Autodesk Inventor part; units mm, degrees
(part 3 of 3)
sketch "Szkic15" plane through (0, 0, 0) normal (0, 0, -1) x (-1, 0, 0)
  line L0 (-9.2546, 25.2956) -> (16.7454, 25.2956) projected
  line L1 (3.7454, 25.2956) -> (3.7525, -18.7044)
  line L2 (-0.9375, -18.7044) -> (8.4425, -18.7044) projected
  circle A0 centre (3.749, 3.2956) radius 15
  line L3 (19.3551, 10.4983) -> (20.5264, 12.5271)
  line L4 (20.5264, 12.5271) -> (22.8692, 12.5271)
  line L5 (22.8692, 12.5271) -> (24.0404, 10.4983)
  line L6 (24.0404, 10.4983) -> (22.8692, 8.4695)
  line L7 (22.8692, 8.4695) -> (20.5264, 8.4695)
  line L8 (20.5264, 8.4695) -> (19.3551, 10.4983)
  line L9 (13.7752, 12.4981) -> (11.4324, 12.4981)
  line L10 (11.4324, 12.4981) -> (10.2611, 10.4693)
  line L11 (10.2611, 10.4693) -> (11.4324, 8.4405)
  line L12 (11.4324, 8.4405) -> (13.7752, 8.4405)
  line L13 (13.7752, 8.4405) -> (14.9464, 10.4693)
  line L14 (14.9464, 10.4693) -> (13.7752, 12.4981)
  line L15 (14.8161, 7.7843) -> (15.9874, 9.8131)
  line L16 (15.9874, 9.8131) -> (18.3302, 9.8131)
  line L17 (18.3302, 9.8131) -> (19.5014, 7.7843)
  line L18 (19.5014, 7.7843) -> (18.3302, 5.7555)
  line L19 (18.3302, 5.7555) -> (15.9874, 5.7555)
  line L20 (15.9874, 5.7555) -> (14.8161, 7.7843)
  line L21 (18.2702, 11.0065) -> (19.4414, 13.0353)
  line L22 (19.4414, 13.0353) -> (18.2702, 15.0641)
  line L23 (18.2702, 15.0641) -> (15.9274, 15.0641)
  line L24 (15.9274, 15.0641) -> (14.7561, 13.0353)
  line L25 (14.7561, 13.0353) -> (15.9274, 11.0065)
  line L26 (15.9274, 11.0065) -> (18.2702, 11.0065)
  line L27 (0.9421, 10.4263) -> (2.1134, 12.4551)
  line L28 (2.1134, 12.4551) -> (4.4562, 12.4551)
  line L29 (4.4562, 12.4551) -> (5.6274, 10.4263)
  line L30 (5.6274, 10.4263) -> (4.4562, 8.3975)
  line L31 (4.4562, 8.3975) -> (2.1134, 8.3975)
  line L32 (2.1134, 8.3975) -> (0.9421, 10.4263)
  line L33 (-3.5969, 7.7123) -> (-2.4256, 9.7411)
  line L34 (-2.4256, 9.7411) -> (-0.0828, 9.7411)
  line L35 (-0.0828, 9.7411) -> (1.0884, 7.7123)
  line L36 (1.0884, 7.7123) -> (-0.0828, 5.6835)
  line L37 (-0.0828, 5.6835) -> (-2.4256, 5.6835)
  line L38 (-2.4256, 5.6835) -> (-3.5969, 7.7123)
  line L39 (2.2234, 7.1181) -> (1.0521, 5.0893)
  line L40 (1.0521, 5.0893) -> (2.2234, 3.0605)
  line L41 (2.2234, 3.0605) -> (4.5662, 3.0605)
  line L42 (4.5662, 3.0605) -> (5.7374, 5.0893)
  line L43 (5.7374, 5.0893) -> (4.5662, 7.1181)
  line L44 (4.5662, 7.1181) -> (2.2234, 7.1181)
  line L45 (-3.3977, 4.9903) -> (-4.5689, 7.0191)
  line L46 (-4.5689, 7.0191) -> (-6.9117, 7.0191)
  line L47 (-6.9117, 7.0191) -> (-8.083, 4.9903)
  line L48 (-8.083, 4.9903) -> (-6.9117, 2.9615)
  line L49 (-6.9117, 2.9615) -> (-4.5689, 2.9615)
  line L50 (-4.5689, 2.9615) -> (-3.3977, 4.9903)
  line L51 (-2.2726, 4.5521) -> (-3.4439, 2.5233)
  line L52 (-3.4439, 2.5233) -> (-2.2726, 0.4945)
  line L53 (-2.2726, 0.4945) -> (0.0702, 0.4945)
  line L54 (0.0702, 0.4945) -> (1.2414, 2.5233)
  line L55 (1.2414, 2.5233) -> (0.0702, 4.5521)
  line L56 (0.0702, 4.5521) -> (-2.2726, 4.5521)
  line L57 (6.6694, 5.7115) -> (9.0122, 5.7115)
  line L58 (9.0122, 5.7115) -> (10.1834, 7.7403)
  line L59 (10.1834, 7.7403) -> (9.0122, 9.7691)
  line L60 (9.0122, 9.7691) -> (6.6694, 9.7691)
  line L61 (6.6694, 9.7691) -> (5.4981, 7.7403)
  line L62 (5.4981, 7.7403) -> (6.6694, 5.7115)
  line L63 (2.2824, 1.8671) -> (1.1111, -0.1617)
  line L64 (1.1111, -0.1617) -> (2.2824, -2.1905)
  line L65 (2.2824, -2.1905) -> (4.6252, -2.1905)
  line L66 (4.6252, -2.1905) -> (5.7964, -0.1617)
  line L67 (5.7964, -0.1617) -> (4.6252, 1.8671)
  line L68 (4.6252, 1.8671) -> (2.2824, 1.8671)
  line L69 (5.6511, 2.5523) -> (6.8224, 4.5811)
  line L70 (6.8224, 4.5811) -> (9.1652, 4.5811)
  line L71 (9.1652, 4.5811) -> (10.3364, 2.5523)
  line L72 (10.3364, 2.5523) -> (9.1652, 0.5235)
  line L73 (9.1652, 0.5235) -> (6.8224, 0.5235)
  line L74 (6.8224, 0.5235) -> (5.6511, 2.5523)
  line L75 (19.4651, 5.1613) -> (20.6364, 7.1901)
  line L76 (20.6364, 7.1901) -> (22.9792, 7.1901)
  line L77 (22.9792, 7.1901) -> (24.1504, 5.1613)
  line L78 (24.1504, 5.1613) -> (22.9792, 3.1325)
  line L79 (22.9792, 3.1325) -> (20.6364, 3.1325)
  line L80 (20.6364, 3.1325) -> (19.4651, 5.1613)
  line L81 (16.1404, 4.6241) -> (14.9691, 2.5953)
  line L82 (14.9691, 2.5953) -> (16.1404, 0.5665)
  line L83 (16.1404, 0.5665) -> (18.4832, 0.5665)
  line L84 (18.4832, 0.5665) -> (19.6544, 2.5953)
  line L85 (19.6544, 2.5953) -> (18.4832, 4.6241)
  line L86 (18.4832, 4.6241) -> (16.1404, 4.6241)
  line L87 (11.3174, 7.1461) -> (10.1461, 5.1173)
  line L88 (10.1461, 5.1173) -> (11.3174, 3.0885)
  line L89 (11.3174, 3.0885) -> (13.6602, 3.0885)
  line L90 (13.6602, 3.0885) -> (14.8314, 5.1173)
  line L91 (14.8314, 5.1173) -> (13.6602, 7.1461)
  line L92 (13.6602, 7.1461) -> (11.3174, 7.1461)
  line L93 (11.3774, 1.8961) -> (10.2061, -0.1327)
  line L94 (10.2061, -0.1327) -> (11.3774, -2.1615)
  line L95 (11.3774, -2.1615) -> (13.7202, -2.1615)
  line L96 (13.7202, -2.1615) -> (14.8914, -0.1327)
  line L97 (14.8914, -0.1327) -> (13.7202, 1.8961)
  line L98 (13.7202, 1.8961) -> (11.3774, 1.8961)
  line L99 (-3.3381, -0.2607) -> (-4.5093, 1.7681)
  line L100 (-4.5093, 1.7681) -> (-6.8521, 1.7681)
  line L101 (-6.8521, 1.7681) -> (-8.0234, -0.2607)
  line L102 (-8.0234, -0.2607) -> (-6.8521, -2.2895)
  line L103 (-6.8521, -2.2895) -> (-4.5093, -2.2895)
  line L104 (-4.5093, -2.2895) -> (-3.3381, -0.2607)
  line L105 (0.1912, -0.9189) -> (-2.1516, -0.9189)
  line L106 (-2.1516, -0.9189) -> (-3.3229, -2.9477)
  line L107 (-3.3229, -2.9477) -> (-2.1516, -4.9765)
  line L108 (-2.1516, -4.9765) -> (0.1912, -4.9765)
  line L109 (0.1912, -4.9765) -> (1.3624, -2.9477)
  line L110 (1.3624, -2.9477) -> (0.1912, -0.9189)
  line L111 (1.2761, -5.4847) -> (2.4474, -3.4559)
  line L112 (2.4474, -3.4559) -> (4.7902, -3.4559)
  line L113 (4.7902, -3.4559) -> (5.9614, -5.4847)
  line L114 (5.9614, -5.4847) -> (4.7902, -7.5135)
  line L115 (4.7902, -7.5135) -> (2.4474, -7.5135)
  line L116 (2.4474, -7.5135) -> (1.2761, -5.4847)
  line L117 (-3.1334, -5.5137) -> (-4.3046, -3.4849)
  line L118 (-4.3046, -3.4849) -> (-6.6474, -3.4849)
  line L119 (-6.6474, -3.4849) -> (-7.8187, -5.5137)
  line L120 (-7.8187, -5.5137) -> (-6.6474, -7.5425)
  line L121 (-6.6474, -7.5425) -> (-4.3046, -7.5425)
  line L122 (-4.3046, -7.5425) -> (-3.1334, -5.5137)
  line L123 (9.2852, -4.9475) -> (10.4564, -2.9187)
  line L124 (10.4564, -2.9187) -> (9.2852, -0.8899)
  line L125 (9.2852, -0.8899) -> (6.9424, -0.8899)
  line L126 (6.9424, -0.8899) -> (5.7711, -2.9187)
  line L127 (5.7711, -2.9187) -> (6.9424, -4.9475)
  line L128 (6.9424, -4.9475) -> (9.2852, -4.9475)
  line L129 (18.6042, -0.8469) -> (16.2614, -0.8469)
  line L130 (16.2614, -0.8469) -> (15.0901, -2.8757)
  line L131 (15.0901, -2.8757) -> (16.2614, -4.9045)
  line L132 (16.2614, -4.9045) -> (18.6042, -4.9045)
  line L133 (18.6042, -4.9045) -> (19.7754, -2.8757)
  line L134 (19.7754, -2.8757) -> (18.6042, -0.8469)
  line L135 (14.1082, -3.4129) -> (11.7654, -3.4129)
  line L136 (11.7654, -3.4129) -> (10.5941, -5.4417)
  line L137 (10.5941, -5.4417) -> (11.7654, -7.4705)
  line L138 (11.7654, -7.4705) -> (14.1082, -7.4705)
  line L139 (14.1082, -7.4705) -> (15.2794, -5.4417)
  line L140 (15.2794, -5.4417) -> (14.1082, -3.4129)
  line L141 (24.2094, -0.0897) -> (23.0382, 1.9391)
  line L142 (23.0382, 1.9391) -> (20.6954, 1.9391)
  line L143 (20.6954, 1.9391) -> (19.5241, -0.0897)
  line L144 (19.5241, -0.0897) -> (20.6954, -2.1185)
  line L145 (20.6954, -2.1185) -> (23.0382, -2.1185)
  line L146 (23.0382, -2.1185) -> (24.2094, -0.0897)
  line L147 (24.1841, -2.8467) -> (25.3554, -0.8179)
  line L148 (25.3554, -0.8179) -> (27.6982, -0.8179)
  line L149 (27.6982, -0.8179) -> (28.8694, -2.8467)
  line L150 (28.8694, -2.8467) -> (27.6982, -4.8755)
  line L151 (27.6982, -4.8755) -> (25.3554, -4.8755)
  line L152 (25.3554, -4.8755) -> (24.1841, -2.8467)
  line L153 (23.2032, -3.3839) -> (20.8604, -3.3839)
  line L154 (20.8604, -3.3839) -> (19.6891, -5.4127)
  line L155 (19.6891, -5.4127) -> (20.8604, -7.4415)
  line L156 (20.8604, -7.4415) -> (23.2032, -7.4415)
  line L157 (23.2032, -7.4415) -> (24.3744, -5.4127)
  line L158 (24.3744, -5.4127) -> (23.2032, -3.3839)
  line L159 (1.3851, -10.8217) -> (2.5564, -8.7929)
  line L160 (2.5564, -8.7929) -> (4.8992, -8.7929)
  line L161 (4.8992, -8.7929) -> (6.0704, -10.8217)
  line L162 (6.0704, -10.8217) -> (4.8992, -12.8505)
  line L163 (4.8992, -12.8505) -> (2.5564, -12.8505)
  line L164 (2.5564, -12.8505) -> (1.3851, -10.8217)
  line L165 (0.4042, -11.3589) -> (-1.9386, -11.3589)
  line L166 (-1.9386, -11.3589) -> (-3.1099, -13.3877)
  line L167 (-3.1099, -13.3877) -> (-1.9386, -15.4165)
  line L168 (-1.9386, -15.4165) -> (0.4042, -15.4165)
  line L169 (0.4042, -15.4165) -> (1.5754, -13.3877)
  line L170 (1.5754, -13.3877) -> (0.4042, -11.3589)
  line L171 (0.2502, -10.2275) -> (1.4214, -8.1987)
  line L172 (1.4214, -8.1987) -> (0.2502, -6.1699)
  line L173 (0.2502, -6.1699) -> (-2.0926, -6.1699)
  line L174 (-2.0926, -6.1699) -> (-3.2639, -8.1987)
  line L175 (-3.2639, -8.1987) -> (-2.0926, -10.2275)
  line L176 (-2.0926, -10.2275) -> (0.2502, -10.2275)
  line L177 (-4.2356, -8.8919) -> (-6.5784, -8.8919)
  line L178 (-6.5784, -8.8919) -> (-7.7497, -10.9207)
  line L179 (-7.7497, -10.9207) -> (-6.5784, -12.9495)
  line L180 (-6.5784, -12.9495) -> (-4.2356, -12.9495)
  line L181 (-4.2356, -12.9495) -> (-3.0644, -10.9207)
  line L182 (-3.0644, -10.9207) -> (-4.2356, -8.8919)
  line L183 (5.8311, -8.1697) -> (7.0024, -6.1409)
  line L184 (7.0024, -6.1409) -> (9.3452, -6.1409)
  line L185 (9.3452, -6.1409) -> (10.5164, -8.1697)
  line L186 (10.5164, -8.1697) -> (9.3452, -10.1985)
  line L187 (9.3452, -10.1985) -> (7.0024, -10.1985)
  line L188 (7.0024, -10.1985) -> (5.8311, -8.1697)
  line L189 (5.9841, -13.3587) -> (7.1554, -11.3299)
  line L190 (7.1554, -11.3299) -> (9.4982, -11.3299)
  line L191 (9.4982, -11.3299) -> (10.6694, -13.3587)
  line L192 (10.6694, -13.3587) -> (9.4982, -15.3875)
  line L193 (9.4982, -15.3875) -> (7.1554, -15.3875)
  line L194 (7.1554, -15.3875) -> (5.9841, -13.3587)
  line L195 (2.6164, -18.1015) -> (4.9592, -18.1015)
  line L196 (4.9592, -18.1015) -> (6.1304, -16.0727)
  line L197 (6.1304, -16.0727) -> (4.9592, -14.0439)
  line L198 (4.9592, -14.0439) -> (2.6164, -14.0439)
  line L199 (2.6164, -14.0439) -> (1.4451, -16.0727)
  line L200 (1.4451, -16.0727) -> (2.6164, -18.1015)
  line L201 (11.6514, -8.7639) -> (10.4801, -10.7927)
  line L202 (10.4801, -10.7927) -> (11.6514, -12.8215)
  line L203 (11.6514, -12.8215) -> (13.9942, -12.8215)
  line L204 (13.9942, -12.8215) -> (15.1654, -10.7927)
  line L205 (15.1654, -10.7927) -> (13.9942, -8.7639)
  line L206 (13.9942, -8.7639) -> (11.6514, -8.7639)
  line L207 (15.3031, -13.3157) -> (16.4744, -11.2869)
  line L208 (16.4744, -11.2869) -> (18.8172, -11.2869)
  line L209 (18.8172, -11.2869) -> (19.9884, -13.3157)
  line L210 (19.9884, -13.3157) -> (18.8172, -15.3445)
  line L211 (18.8172, -15.3445) -> (16.4744, -15.3445)
  line L212 (16.4744, -15.3445) -> (15.3031, -13.3157)
  line L213 (15.1491, -8.1267) -> (16.3204, -6.0979)
  line L214 (16.3204, -6.0979) -> (18.6632, -6.0979)
  line L215 (18.6632, -6.0979) -> (19.8344, -8.1267)
  line L216 (19.8344, -8.1267) -> (18.6632, -10.1555)
  line L217 (18.6632, -10.1555) -> (16.3204, -10.1555)
  line L218 (16.3204, -10.1555) -> (15.1491, -8.1267)
  line L219 (19.7981, -10.7497) -> (20.9694, -8.7209)
  line L220 (20.9694, -8.7209) -> (23.3122, -8.7209)
  line L221 (23.3122, -8.7209) -> (24.4834, -10.7497)
  line L222 (24.4834, -10.7497) -> (23.3122, -12.7785)
  line L223 (23.3122, -12.7785) -> (20.9694, -12.7785)
  line L224 (20.9694, -12.7785) -> (19.7981, -10.7497)
  line L225 (25.4154, -10.1265) -> (27.7582, -10.1265)
  line L226 (27.7582, -10.1265) -> (28.9294, -8.0977)
  line L227 (28.9294, -8.0977) -> (27.7582, -6.0689)
  line L228 (27.7582, -6.0689) -> (25.4154, -6.0689)
  line L229 (25.4154, -6.0689) -> (24.2441, -8.0977)
  line L230 (24.2441, -8.0977) -> (25.4154, -10.1265)
  line L231 (25.5684, -11.2579) -> (24.3971, -13.2867)
  line L232 (24.3971, -13.2867) -> (25.5684, -15.3155)
  line L233 (25.5684, -15.3155) -> (27.9112, -15.3155)
  line L234 (27.9112, -15.3155) -> (29.0824, -13.2867)
  line L235 (29.0824, -13.2867) -> (27.9112, -11.2579)
  line L236 (27.9112, -11.2579) -> (25.5684, -11.2579)
  line L237 (11.7104, -18.0725) -> (14.0532, -18.0725)
  line L238 (14.0532, -18.0725) -> (15.2244, -16.0437)
  line L239 (15.2244, -16.0437) -> (14.0532, -14.0149)
  line L240 (14.0532, -14.0149) -> (11.7104, -14.0149)
  line L241 (11.7104, -14.0149) -> (10.5391, -16.0437)
  line L242 (10.5391, -16.0437) -> (11.7104, -18.0725)
  line L243 (21.0294, -13.9719) -> (19.8581, -16.0007)
  line L244 (19.8581, -16.0007) -> (21.0294, -18.0295)
  line L245 (21.0294, -18.0295) -> (23.3722, -18.0295)
  line L246 (23.3722, -18.0295) -> (24.5434, -16.0007)
  line L247 (24.5434, -16.0007) -> (23.3722, -13.9719)
  line L248 (23.3722, -13.9719) -> (21.0294, -13.9719)
  line L249 (-26.4363, -0.3327) -> (-25.265, 1.6961)
  line L250 (-25.265, 1.6961) -> (-22.9222, 1.6961)
  line L251 (-22.9222, 1.6961) -> (-21.751, -0.3327)
  line L252 (-21.751, -0.3327) -> (-22.9222, -2.3615)
  line L253 (-22.9222, -2.3615) -> (-25.265, -2.3615)
  line L254 (-25.265, -2.3615) -> (-26.4363, -0.3327)
  line L255 (-18.0387, -1.0469) -> (-20.3815, -1.0469)
  line L256 (-20.3815, -1.0469) -> (-21.5528, -3.0757)
  line L257 (-21.5528, -3.0757) -> (-20.3815, -5.1045)
  line L258 (-20.3815, -5.1045) -> (-18.0387, -5.1045)
  line L259 (-18.0387, -5.1045) -> (-16.8675, -3.0757)
  line L260 (-16.8675, -3.0757) -> (-18.0387, -1.0469)
  line L261 (-22.5341, -3.6119) -> (-24.8769, -3.6119)
  line L262 (-24.8769, -3.6119) -> (-26.0482, -5.6407)
  line L263 (-26.0482, -5.6407) -> (-24.8769, -7.6695)
  line L264 (-24.8769, -7.6695) -> (-22.5341, -7.6695)
  line L265 (-22.5341, -7.6695) -> (-21.3629, -5.6407)
  line L266 (-21.3629, -5.6407) -> (-22.5341, -3.6119)
  line L267 (-27.357, -1.0899) -> (-29.6998, -1.0899)
  line L268 (-29.6998, -1.0899) -> (-30.8711, -3.1187)
  line L269 (-30.8711, -3.1187) -> (-29.6998, -5.1475)
  line L270 (-29.6998, -5.1475) -> (-27.357, -5.1475)
  line L271 (-27.357, -5.1475) -> (-26.1858, -3.1187)
  line L272 (-26.1858, -3.1187) -> (-27.357, -1.0899)
  line L273 (-16.9536, -5.6127) -> (-15.7823, -3.5839)
  line L274 (-15.7823, -3.5839) -> (-13.4395, -3.5839)
  line L275 (-13.4395, -3.5839) -> (-12.2683, -5.6127)
  line L276 (-12.2683, -5.6127) -> (-13.4395, -7.6415)
  line L277 (-13.4395, -7.6415) -> (-15.7823, -7.6415)
  line L278 (-15.7823, -7.6415) -> (-16.9536, -5.6127)
  line L279 (-27.4773, 0.3235) -> (-26.3061, 2.3523)
  line L280 (-26.3061, 2.3523) -> (-27.4773, 4.3811)
  line L281 (-27.4773, 4.3811) -> (-29.8201, 4.3811)
  line L282 (-29.8201, 4.3811) -> (-30.9914, 2.3523)
  line L283 (-30.9914, 2.3523) -> (-29.8201, 0.3235)
  line L284 (-29.8201, 0.3235) -> (-27.4773, 0.3235)
  line L285 (-30.8115, -8.3697) -> (-29.6402, -6.3409)
  line L286 (-29.6402, -6.3409) -> (-27.2974, -6.3409)
  line L287 (-27.2974, -6.3409) -> (-26.1262, -8.3697)
  line L288 (-26.1262, -8.3697) -> (-27.2974, -10.3985)
  line L289 (-27.2974, -10.3985) -> (-29.6402, -10.3985)
  line L290 (-29.6402, -10.3985) -> (-30.8115, -8.3697)
  line L291 (-21.4931, -8.3257) -> (-20.3218, -6.2969)
  line L292 (-20.3218, -6.2969) -> (-17.979, -6.2969)
  line L293 (-17.979, -6.2969) -> (-16.8078, -8.3257)
  line L294 (-16.8078, -8.3257) -> (-17.979, -10.3545)
  line L295 (-17.979, -10.3545) -> (-20.3218, -10.3545)
  line L296 (-20.3218, -10.3545) -> (-21.4931, -8.3257)
  line L297 (-21.3397, -13.5147) -> (-20.1684, -11.4859)
  line L298 (-20.1684, -11.4859) -> (-17.8256, -11.4859)
  line L299 (-17.8256, -11.4859) -> (-16.6544, -13.5147)
  line L300 (-16.6544, -13.5147) -> (-17.8256, -15.5435)
  line L301 (-17.8256, -15.5435) -> (-20.1684, -15.5435)
  line L302 (-20.1684, -15.5435) -> (-21.3397, -13.5147)
  line L303 (-22.6485, -8.9639) -> (-24.9913, -8.9639)
  line L304 (-24.9913, -8.9639) -> (-26.1626, -10.9927)
  line L305 (-26.1626, -10.9927) -> (-24.9913, -13.0215)
  line L306 (-24.9913, -13.0215) -> (-22.6485, -13.0215)
  line L307 (-22.6485, -13.0215) -> (-21.4773, -10.9927)
  line L308 (-21.4773, -10.9927) -> (-22.6485, -8.9639)
  line L309 (-27.1439, -11.5299) -> (-29.4867, -11.5299)
  line L310 (-29.4867, -11.5299) -> (-30.658, -13.5587)
  line L311 (-30.658, -13.5587) -> (-29.4867, -15.5875)
  line L312 (-29.4867, -15.5875) -> (-27.1439, -15.5875)
  line L313 (-27.1439, -15.5875) -> (-25.9727, -13.5587)
  line L314 (-25.9727, -13.5587) -> (-27.1439, -11.5299)
  line L315 (-24.9317, -14.2149) -> (-26.103, -16.2437)
  line L316 (-26.103, -16.2437) -> (-24.9317, -18.2725)
  line L317 (-24.9317, -18.2725) -> (-22.5889, -18.2725)
  line L318 (-22.5889, -18.2725) -> (-21.4177, -16.2437)
  line L319 (-21.4177, -16.2437) -> (-22.5889, -14.2149)
  line L320 (-22.5889, -14.2149) -> (-24.9317, -14.2149)
  line L321 (-30.5719, -11.0217) -> (-31.7431, -8.9929)
  line L322 (-31.7431, -8.9929) -> (-34.0859, -8.9929)
  line L323 (-34.0859, -8.9929) -> (-35.2572, -11.0217)
  line L324 (-35.2572, -11.0217) -> (-34.0859, -13.0505)
  line L325 (-34.0859, -13.0505) -> (-31.7431, -13.0505)
  line L326 (-31.7431, -13.0505) -> (-30.5719, -11.0217)
  line L327 (-31.6835, -14.2429) -> (-34.0263, -14.2429)
  line L328 (-34.0263, -14.2429) -> (-35.1976, -16.2717)
  line L329 (-35.1976, -16.2717) -> (-34.0263, -18.3005)
  line L330 (-34.0263, -18.3005) -> (-31.6835, -18.3005)
  line L331 (-31.6835, -18.3005) -> (-30.5123, -16.2717)
  line L332 (-30.5123, -16.2717) -> (-31.6835, -14.2429)
  line L333 (-9.3542, 16.3825) -> (-8.183, 18.4113)
  line L334 (-8.183, 18.4113) -> (-9.3542, 20.4401)
  line L335 (-9.3542, 20.4401) -> (-11.697, 20.4401)
  line L336 (-11.697, 20.4401) -> (-12.8683, 18.4113)
  line L337 (-12.8683, 18.4113) -> (-11.697, 16.3825)
  line L338 (-11.697, 16.3825) -> (-9.3542, 16.3825)
  line L339 (-17.2869, 10.2983) -> (-16.1156, 12.3271)
  line L340 (-16.1156, 12.3271) -> (-13.7728, 12.3271)
  line L341 (-13.7728, 12.3271) -> (-12.6016, 10.2983)
  line L342 (-12.6016, 10.2983) -> (-13.7728, 8.2695)
  line L343 (-13.7728, 8.2695) -> (-16.1156, 8.2695)
  line L344 (-16.1156, 8.2695) -> (-17.2869, 10.2983)
  line L345 (-13.0218, 23.6003) -> (-11.8505, 21.5715)
  line L346 (-11.8505, 21.5715) -> (-9.5077, 21.5715)
  line L347 (-9.5077, 21.5715) -> (-8.3365, 23.6003)
  line L348 (-8.3365, 23.6003) -> (-9.5077, 25.6291)
  line L349 (-9.5077, 25.6291) -> (-11.8505, 25.6291)
  line L350 (-11.8505, 25.6291) -> (-13.0218, 23.6003)
  line L351 (-13.0218, 23.6003) -> (-11.8505, 21.5715)
  line L352 (-16.8443, -10.9487) -> (-15.673, -8.9199)
  line L353 (-15.673, -8.9199) -> (-13.3302, -8.9199)
  line L354 (-13.3302, -8.9199) -> (-12.159, -10.9487)
  line L355 (-12.159, -10.9487) -> (-13.3302, -12.9775)
  line L356 (-13.3302, -12.9775) -> (-15.673, -12.9775)
  line L357 (-15.673, -12.9775) -> (-16.8443, -10.9487)
  line L358 (-11.5606, 5.5845) -> (-9.2178, 5.5845)
  line L359 (-9.2178, 5.5845) -> (-8.0466, 7.6133)
  line L360 (-8.0466, 7.6133) -> (-9.2178, 9.6421)
  line L361 (-9.2178, 9.6421) -> (-11.5606, 9.6421)
  line L362 (-11.5606, 9.6421) -> (-12.7319, 7.6133)
  line L363 (-12.7319, 7.6133) -> (-11.5606, 5.5845)
  line L364 (-12.5785, 2.4243) -> (-11.4072, 4.4531)
  line L365 (-11.4072, 4.4531) -> (-9.0644, 4.4531)
  line L366 (-9.0644, 4.4531) -> (-7.8932, 2.4243)
  line L367 (-7.8932, 2.4243) -> (-9.0644, 0.3955)
  line L368 (-9.0644, 0.3955) -> (-11.4072, 0.3955)
  line L369 (-11.4072, 0.3955) -> (-12.5785, 2.4243)
  line L370 (-13.6635, 2.9325) -> (-12.4923, 4.9613)
  line L371 (-12.4923, 4.9613) -> (-13.6635, 6.9901)
  line L372 (-13.6635, 6.9901) -> (-16.0063, 6.9901)
  line L373 (-16.0063, 6.9901) -> (-17.1776, 4.9613)
  line L374 (-17.1776, 4.9613) -> (-16.0063, 2.9325)
  line L375 (-16.0063, 2.9325) -> (-13.6635, 2.9325)
  line L376 (-12.2451, -13.4857) -> (-11.0738, -11.4569)
  line L377 (-11.0738, -11.4569) -> (-8.731, -11.4569)
  line L378 (-8.731, -11.4569) -> (-7.5598, -13.4857)
  line L379 (-7.5598, -13.4857) -> (-8.731, -15.5145)
  line L380 (-8.731, -15.5145) -> (-11.0738, -15.5145)
  line L381 (-11.0738, -15.5145) -> (-12.2451, -13.4857)
  line L382 (-15.6134, -18.2285) -> (-13.2706, -18.2285)
  line L383 (-13.2706, -18.2285) -> (-12.0994, -16.1997)
  line L384 (-12.0994, -16.1997) -> (-13.2706, -14.1709)
  line L385 (-13.2706, -14.1709) -> (-15.6134, -14.1709)
  line L386 (-15.6134, -14.1709) -> (-16.7847, -16.1997)
  line L387 (-16.7847, -16.1997) -> (-15.6134, -18.2285)
  line L388 (-7.6901, -16.1717) -> (-6.5188, -14.1429)
  line L389 (-6.5188, -14.1429) -> (-4.176, -14.1429)
  line L390 (-4.176, -14.1429) -> (-3.0048, -16.1717)
  line L391 (-3.0048, -16.1717) -> (-4.176, -18.2005)
  line L392 (-4.176, -18.2005) -> (-6.5188, -18.2005)
  line L393 (-6.5188, -18.2005) -> (-7.6901, -16.1717)
  line L394 (-8.9441, -1.0179) -> (-11.2869, -1.0179)
  line L395 (-11.2869, -1.0179) -> (-12.4582, -3.0467)
  line L396 (-12.4582, -3.0467) -> (-11.2869, -5.0755)
  line L397 (-11.2869, -5.0755) -> (-8.9441, -5.0755)
  line L398 (-8.9441, -5.0755) -> (-7.7729, -3.0467)
  line L399 (-7.7729, -3.0467) -> (-8.9441, -1.0179)
  line L400 (-12.3986, -8.2977) -> (-11.2273, -6.2689)
  line L401 (-11.2273, -6.2689) -> (-8.8845, -6.2689)
  line L402 (-8.8845, -6.2689) -> (-7.7133, -8.2977)
  line L403 (-7.7133, -8.2977) -> (-8.8845, -10.3265)
  line L404 (-8.8845, -10.3265) -> (-11.2273, -10.3265)
  line L405 (-11.2273, -10.3265) -> (-12.3986, -8.2977)
  line L406 (-4.7992, 13.6975) -> (-3.628, 15.7263)
  line L407 (-3.628, 15.7263) -> (-4.7992, 17.7551)
  line L408 (-4.7992, 17.7551) -> (-7.142, 17.7551)
  line L409 (-7.142, 17.7551) -> (-8.3133, 15.7263)
  line L410 (-8.3133, 15.7263) -> (-7.142, 13.6975)
  line L411 (-7.142, 13.6975) -> (-4.7992, 13.6975)
  line L412 (-8.152, 10.3973) -> (-6.9807, 12.4261)
  line L413 (-6.9807, 12.4261) -> (-4.6379, 12.4261)
  line L414 (-4.6379, 12.4261) -> (-3.4667, 10.3973)
  line L415 (-3.4667, 10.3973) -> (-4.6379, 8.3685)
  line L416 (-4.6379, 8.3685) -> (-6.9807, 8.3685)
  line L417 (-6.9807, 8.3685) -> (-8.152, 10.3973)
  line L418 (-12.4327, -0.2897) -> (-13.6039, 1.7391)
  line L419 (-13.6039, 1.7391) -> (-15.9467, 1.7391)
  line L420 (-15.9467, 1.7391) -> (-17.118, -0.2897)
  line L421 (-17.118, -0.2897) -> (-15.9467, -2.3185)
  line L422 (-15.9467, -2.3185) -> (-13.6039, -2.3185)
  line L423 (-13.6039, -2.3185) -> (-12.4327, -0.2897)
  line L424 (14.5261, 23.7703) -> (15.6974, 25.7991)
  line L425 (15.6974, 25.7991) -> (18.0402, 25.7991)
  line L426 (18.0402, 25.7991) -> (19.2114, 23.7703)
  line L427 (19.2114, 23.7703) -> (18.0402, 21.7415)
  line L428 (18.0402, 21.7415) -> (15.6974, 21.7415)
  line L429 (15.6974, 21.7415) -> (14.5261, 23.7703)
  line L430 (25.0224, 15.0921) -> (23.8511, 13.0633)
  line L431 (23.8511, 13.0633) -> (25.0224, 11.0345)
  line L432 (25.0224, 11.0345) -> (27.3652, 11.0345)
  line L433 (27.3652, 11.0345) -> (28.5364, 13.0633)
  line L434 (28.5364, 13.0633) -> (27.3652, 15.0921)
  line L435 (27.3652, 15.0921) -> (25.0224, 15.0921)
  line L436 (29.5514, 12.5511) -> (28.3801, 10.5223)
  line L437 (28.3801, 10.5223) -> (29.5514, 8.4935)
  line L438 (29.5514, 8.4935) -> (31.8942, 8.4935)
  line L439 (31.8942, 8.4935) -> (33.0654, 10.5223)
  line L440 (33.0654, 10.5223) -> (31.8942, 12.5511)
  line L441 (31.8942, 12.5511) -> (29.5514, 12.5511)
  line L442 (37.5604, 13.0883) -> (36.3892, 15.1171)
  line L443 (36.3892, 15.1171) -> (34.0464, 15.1171)
  line L444 (34.0464, 15.1171) -> (32.8751, 13.0883)
  line L445 (32.8751, 13.0883) -> (34.0464, 11.0595)
  line L446 (34.0464, 11.0595) -> (36.3892, 11.0595)
  line L447 (36.3892, 11.0595) -> (37.5604, 13.0883)
  line L448 (15.8504, 20.6111) -> (14.6791, 18.5823)
  line L449 (14.6791, 18.5823) -> (15.8504, 16.5535)
  line L450 (15.8504, 16.5535) -> (18.1932, 16.5535)
  line L451 (18.1932, 16.5535) -> (19.3644, 18.5823)
  line L452 (19.3644, 18.5823) -> (18.1932, 20.6111)
  line L453 (18.1932, 20.6111) -> (15.8504, 20.6111)
  line L454 (32.9351, 7.8373) -> (34.1064, 9.8661)
  line L455 (34.1064, 9.8661) -> (36.4492, 9.8661)
  line L456 (36.4492, 9.8661) -> (37.6204, 7.8373)
  line L457 (37.6204, 7.8373) -> (36.4492, 5.8085)
  line L458 (36.4492, 5.8085) -> (34.1064, 5.8085)
  line L459 (34.1064, 5.8085) -> (32.9351, 7.8373)
  line L460 (32.0732, 7.2191) -> (29.7304, 7.2191)
  line L461 (29.7304, 7.2191) -> (28.5591, 5.1903)
  line L462 (28.5591, 5.1903) -> (29.7304, 3.1615)
  line L463 (29.7304, 3.1615) -> (32.0732, 3.1615)
  line L464 (32.0732, 3.1615) -> (33.2444, 5.1903)
  line L465 (33.2444, 5.1903) -> (32.0732, 7.2191)
  line L466 (32.1332, 1.9681) -> (29.7904, 1.9681)
  line L467 (29.7904, 1.9681) -> (28.6191, -0.0607)
  line L468 (28.6191, -0.0607) -> (29.7904, -2.0895)
  line L469 (29.7904, -2.0895) -> (32.1332, -2.0895)
  line L470 (32.1332, -2.0895) -> (33.3044, -0.0607)
  line L471 (33.3044, -0.0607) -> (32.1332, 1.9681)
  line L472 (33.0881, 2.6493) -> (34.2594, 4.6781)
  line L473 (34.2594, 4.6781) -> (36.6022, 4.6781)
  line L474 (36.6022, 4.6781) -> (37.7734, 2.6493)
  line L475 (37.7734, 2.6493) -> (36.6022, 0.6205)
  line L476 (36.6022, 0.6205) -> (34.2594, 0.6205)
  line L477 (34.2594, 0.6205) -> (33.0881, 2.6493)
  line L478 (24.0641, 2.6243) -> (25.2354, 4.6531)
  line L479 (25.2354, 4.6531) -> (27.5782, 4.6531)
  line L480 (27.5782, 4.6531) -> (28.7494, 2.6243)
  line L481 (28.7494, 2.6243) -> (27.5782, 0.5955)
  line L482 (27.5782, 0.5955) -> (25.2354, 0.5955)
  line L483 (25.2354, 0.5955) -> (24.0641, 2.6243)
  line L484 (30.1234, -18.0005) -> (32.4662, -18.0005)
  line L485 (32.4662, -18.0005) -> (33.6374, -15.9717)
  line L486 (33.6374, -15.9717) -> (32.4662, -13.9429)
  line L487 (32.4662, -13.9429) -> (30.1234, -13.9429)
  line L488 (30.1234, -13.9429) -> (28.9521, -15.9717)
  line L489 (28.9521, -15.9717) -> (30.1234, -18.0005)
  line L490 (28.7131, -5.3877) -> (29.8844, -3.3589)
  line L491 (29.8844, -3.3589) -> (32.2272, -3.3589)
  line L492 (32.2272, -3.3589) -> (33.3984, -5.3877)
  line L493 (33.3984, -5.3877) -> (32.2272, -7.4165)
  line L494 (32.2272, -7.4165) -> (29.8844, -7.4165)
  line L495 (29.8844, -7.4165) -> (28.7131, -5.3877)
  line L496 (32.4072, -12.7495) -> (33.5784, -10.7207)
  line L497 (33.5784, -10.7207) -> (32.4072, -8.6919)
  line L498 (32.4072, -8.6919) -> (30.0644, -8.6919)
  line L499 (30.0644, -8.6919) -> (28.8931, -10.7207)
  line L500 (28.8931, -10.7207) -> (30.0644, -12.7495)
  line L501 (30.0644, -12.7495) -> (32.4072, -12.7495)
  line L502 (23.9101, 7.8133) -> (25.0814, 9.8421)
  line L503 (25.0814, 9.8421) -> (27.4242, 9.8421)
  line L504 (27.4242, 9.8421) -> (28.5954, 7.8133)
  line L505 (28.5954, 7.8133) -> (27.4242, 5.7845)
  line L506 (27.4242, 5.7845) -> (25.0814, 5.7845)
  line L507 (25.0814, 5.7845) -> (23.9101, 7.8133)
  line L508 (33.2681, -8.0727) -> (34.4394, -6.0439)
  line L509 (34.4394, -6.0439) -> (36.7822, -6.0439)
  line L510 (36.7822, -6.0439) -> (37.9534, -8.0727)
  line L511 (37.9534, -8.0727) -> (36.7822, -10.1015)
  line L512 (36.7822, -10.1015) -> (34.4394, -10.1015)
  line L513 (34.4394, -10.1015) -> (33.2681, -8.0727)
  line L514 (34.5934, -11.2329) -> (33.4221, -13.2617)
  line L515 (33.4221, -13.2617) -> (34.5934, -15.2905)
  line L516 (34.5934, -15.2905) -> (36.9362, -15.2905)
  line L517 (36.9362, -15.2905) -> (38.1074, -13.2617)
  line L518 (38.1074, -13.2617) -> (36.9362, -11.2329)
  line L519 (36.9362, -11.2329) -> (34.5934, -11.2329)
  line L520 (33.2091, -2.8227) -> (34.3804, -0.7939)
  line L521 (34.3804, -0.7939) -> (36.7232, -0.7939)
  line L522 (36.7232, -0.7939) -> (37.8944, -2.8227)
  line L523 (37.8944, -2.8227) -> (36.7232, -4.8515)
  line L524 (36.7232, -4.8515) -> (34.3804, -4.8515)
  line L525 (34.3804, -4.8515) -> (33.2091, -2.8227)
  line L526 (4.3362, 13.7955) -> (5.5074, 15.8243)
  line L527 (5.5074, 15.8243) -> (4.3362, 17.8531)
  line L528 (4.3362, 17.8531) -> (1.9934, 17.8531)
  line L529 (1.9934, 17.8531) -> (0.8221, 15.8243)
  line L530 (0.8221, 15.8243) -> (1.9934, 13.7955)
  line L531 (1.9934, 13.7955) -> (4.3362, 13.7955)
  line L532 (10.1234, 12.9913) -> (8.9522, 15.0201)
  line L533 (8.9522, 15.0201) -> (6.6094, 15.0201)
  line L534 (6.6094, 15.0201) -> (5.4381, 12.9913)
  line L535 (5.4381, 12.9913) -> (6.6094, 10.9625)
  line L536 (6.6094, 10.9625) -> (8.9522, 10.9625)
  line L537 (8.9522, 10.9625) -> (10.1234, 12.9913)
  line L538 (-3.7339, 18.5103) -> (-2.5626, 20.5391)
  line L539 (-2.5626, 20.5391) -> (-0.2198, 20.5391)
  line L540 (-0.2198, 20.5391) -> (0.9514, 18.5103)
  line L541 (0.9514, 18.5103) -> (-0.2198, 16.4815)
  line L542 (-0.2198, 16.4815) -> (-2.5626, 16.4815)
  line L543 (-2.5626, 16.4815) -> (-3.7339, 18.5103)
  line L544 (-0.1428, 14.9921) -> (-2.4856, 14.9921)
  line L545 (-2.4856, 14.9921) -> (-3.6569, 12.9633)
  line L546 (-3.6569, 12.9633) -> (-2.4856, 10.9345)
  line L547 (-2.4856, 10.9345) -> (-0.1428, 10.9345)
  line L548 (-0.1428, 10.9345) -> (1.0284, 12.9633)
  line L549 (1.0284, 12.9633) -> (-0.1428, 14.9921)
  line L550 (10.0464, 18.5383) -> (8.8752, 20.5671)
  line L551 (8.8752, 20.5671) -> (6.5324, 20.5671)
  line L552 (6.5324, 20.5671) -> (5.3611, 18.5383)
  line L553 (5.3611, 18.5383) -> (6.5324, 16.5095)
  line L554 (6.5324, 16.5095) -> (8.8752, 16.5095)
  line L555 (8.8752, 16.5095) -> (10.0464, 18.5383)
  line L556 (9.8571, 21.1043) -> (11.0284, 23.1331)
  line L557 (11.0284, 23.1331) -> (13.3712, 23.1331)
  line L558 (13.3712, 23.1331) -> (14.5424, 21.1043)
  line L559 (14.5424, 21.1043) -> (13.3712, 19.0755)
  line L560 (13.3712, 19.0755) -> (11.0284, 19.0755)
  line L561 (11.0284, 19.0755) -> (9.8571, 21.1043)
  line L562 (9.9161, 15.8533) -> (11.0874, 17.8821)
  line L563 (11.0874, 17.8821) -> (13.4302, 17.8821)
  line L564 (13.4302, 17.8821) -> (14.6014, 15.8533)
  line L565 (14.6014, 15.8533) -> (13.4302, 13.8245)
  line L566 (13.4302, 13.8245) -> (11.0874, 13.8245)
  line L567 (11.0874, 13.8245) -> (9.9161, 15.8533)
  line L568 (-0.3728, 21.6695) -> (0.7984, 23.6983)
  line L569 (0.7984, 23.6983) -> (-0.3728, 25.7271)
  line L570 (-0.3728, 25.7271) -> (-2.7156, 25.7271)
  line L571 (-2.7156, 25.7271) -> (-3.8869, 23.6983)
  line L572 (-3.8869, 23.6983) -> (-2.7156, 21.6695)
  line L573 (-2.7156, 21.6695) -> (-0.3728, 21.6695)
  line L574 (1.9334, 19.0465) -> (4.2762, 19.0465)
  line L575 (4.2762, 19.0465) -> (5.4474, 21.0753)
  line L576 (5.4474, 21.0753) -> (4.2762, 23.1041)
  line L577 (4.2762, 23.1041) -> (1.9334, 23.1041)
  line L578 (1.9334, 23.1041) -> (0.7621, 21.0753)
  line L579 (0.7621, 21.0753) -> (1.9334, 19.0465)
  line L580 (8.7222, 21.6985) -> (9.8934, 23.7273)
  line L581 (9.8934, 23.7273) -> (8.7222, 25.7561)
  line L582 (8.7222, 25.7561) -> (6.3794, 25.7561)
  line L583 (6.3794, 25.7561) -> (5.2081, 23.7273)
  line L584 (5.2081, 23.7273) -> (6.3794, 21.6985)
  line L585 (6.3794, 21.6985) -> (8.7222, 21.6985)
  line L586 (-3.6876, 20.9773) -> (-4.8588, 23.0061)
  line L587 (-4.8588, 23.0061) -> (-7.2016, 23.0061)
  line L588 (-7.2016, 23.0061) -> (-8.3729, 20.9773)
  line L589 (-8.3729, 20.9773) -> (-7.2016, 18.9485)
  line L590 (-7.2016, 18.9485) -> (-4.8588, 18.9485)
  line L591 (-4.8588, 18.9485) -> (-3.6876, 20.9773)
  line L592 (-22.8674, 12.2981) -> (-25.2102, 12.2981)
  line L593 (-25.2102, 12.2981) -> (-26.3815, 10.2693)
  line L594 (-26.3815, 10.2693) -> (-25.2102, 8.2405)
  line L595 (-25.2102, 8.2405) -> (-22.8674, 8.2405)
  line L596 (-22.8674, 8.2405) -> (-21.6962, 10.2693)
  line L597 (-21.6962, 10.2693) -> (-22.8674, 12.2981)
  line L598 (-20.5017, 4.4251) -> (-21.673, 2.3963)
  line L599 (-21.673, 2.3963) -> (-20.5017, 0.3675)
  line L600 (-20.5017, 0.3675) -> (-18.1589, 0.3675)
  line L601 (-18.1589, 0.3675) -> (-16.9877, 2.3963)
  line L602 (-16.9877, 2.3963) -> (-18.1589, 4.4251)
  line L603 (-18.1589, 4.4251) -> (-20.5017, 4.4251)
  line L604 (-20.6552, 9.6131) -> (-21.8265, 7.5843)
  line L605 (-21.8265, 7.5843) -> (-20.6552, 5.5555)
  line L606 (-20.6552, 5.5555) -> (-18.3124, 5.5555)
  line L607 (-18.3124, 5.5555) -> (-17.1412, 7.5843)
  line L608 (-17.1412, 7.5843) -> (-18.3124, 9.6131)
  line L609 (-18.3124, 9.6131) -> (-20.6552, 9.6131)
  line L610 (-22.9819, 6.9471) -> (-25.3247, 6.9471)
  line L611 (-25.3247, 6.9471) -> (-26.496, 4.9183)
  line L612 (-26.496, 4.9183) -> (-25.3247, 2.8895)
  line L613 (-25.3247, 2.8895) -> (-22.9819, 2.8895)
  line L614 (-22.9819, 2.8895) -> (-21.8107, 4.9183)
  line L615 (-21.8107, 4.9183) -> (-22.9819, 6.9471)
  line L616 (-29.9735, 9.5701) -> (-31.1448, 7.5413)
  line L617 (-31.1448, 7.5413) -> (-29.9735, 5.5125)
  line L618 (-29.9735, 5.5125) -> (-27.6307, 5.5125)
  line L619 (-27.6307, 5.5125) -> (-26.4595, 7.5413)
  line L620 (-26.4595, 7.5413) -> (-27.6307, 9.5701)
  line L621 (-27.6307, 9.5701) -> (-29.9735, 9.5701)
  line L622 (-27.6903, 10.7635) -> (-26.5191, 12.7923)
  line L623 (-26.5191, 12.7923) -> (-27.6903, 14.8211)
  line L624 (-27.6903, 14.8211) -> (-30.0331, 14.8211)
  line L625 (-30.0331, 14.8211) -> (-31.2044, 12.7923)
  line L626 (-31.2044, 12.7923) -> (-30.0331, 10.7635)
  line L627 (-30.0331, 10.7635) -> (-27.6903, 10.7635)
  line L628 (-20.7148, 14.8641) -> (-21.8861, 12.8353)
  line L629 (-21.8861, 12.8353) -> (-20.7148, 10.8065)
  line L630 (-20.7148, 10.8065) -> (-18.372, 10.8065)
  line L631 (-18.372, 10.8065) -> (-17.2008, 12.8353)
  line L632 (-17.2008, 12.8353) -> (-18.372, 14.8641)
  line L633 (-18.372, 14.8641) -> (-20.7148, 14.8641)
  line L634 (-3.0329, -18.9347) -> (-1.8616, -16.9059)
  line L635 (-1.8616, -16.9059) -> (0.4812, -16.9059)
  line L636 (0.4812, -16.9059) -> (1.6524, -18.9347)
  line L637 (6.0611, -18.9057) -> (7.2324, -16.8769)
  line L638 (7.2324, -16.8769) -> (9.5752, -16.8769)
  line L639 (9.5752, -16.8769) -> (10.7464, -18.9057)
  line L640 (15.3791, -18.8627) -> (16.5504, -16.8339)
  line L641 (16.5504, -16.8339) -> (18.8932, -16.8339)
  line L642 (18.8932, -16.8339) -> (20.0644, -18.8627)
  line L643 (-32.0168, 1.6671) -> (-30.8456, -0.3617)
  line L644 (-30.8456, -0.3617) -> (-32.0168, -2.3905)
  line L645 (-31.8524, -3.6559) -> (-30.6812, -5.6847)
  line L646 (-30.6812, -5.6847) -> (-31.8524, -7.7135)
  line L647 (-31.8524, -7.7135) -> (-34.1952, -7.7135)
  line L648 (-36.2385, -11.5579) -> (-35.0673, -13.5867)
  line L649 (-35.0673, -13.5867) -> (-36.2385, -15.6155)
  line L650 (-21.2629, -19.0617) -> (-20.0916, -17.0329)
  line L651 (-20.0916, -17.0329) -> (-17.7488, -17.0329)
  line L652 (-17.7488, -17.0329) -> (-16.5776, -19.0617)
  line L653 (-30.5812, -19.1057) -> (-29.4099, -17.0769)
  line L654 (-29.4099, -17.0769) -> (-27.0671, -17.0769)
  line L655 (-27.0671, -17.0769) -> (-25.8959, -19.1057)
  line L656 (-13.8938, 17.7261) -> (-12.7226, 15.6973)
  line L657 (-12.7226, 15.6973) -> (-13.8938, 13.6685)
  line L658 (-13.8938, 13.6685) -> (-16.2366, 13.6685)
  line L659 (-16.2366, 13.6685) -> (-17.4079, 15.6973)
  line L660 (-12.1683, -19.0327) -> (-10.997, -17.0039)
  line L661 (-10.997, -17.0039) -> (-8.6542, -17.0039)
  line L662 (-8.6542, -17.0039) -> (-7.483, -19.0327)
  line L663 (20.3464, 19.1185) -> (19.1751, 21.1473)
  line L664 (19.1751, 21.1473) -> (20.3464, 23.1761)
  line L665 (33.0144, 15.9253) -> (31.8432, 13.8965)
  line L666 (31.8432, 13.8965) -> (29.5004, 13.8965)
  line L667 (29.5004, 13.8965) -> (28.3291, 15.9253)
  line L668 (23.9194, 15.8973) -> (22.7482, 13.8685)
  line L669 (22.7482, 13.8685) -> (20.4054, 13.8685)
  line L670 (20.4054, 13.8685) -> (19.2341, 15.8973)
  line L671 (19.2341, 15.8973) -> (20.4054, 17.9261)
  line L672 (38.6464, 8.5225) -> (37.4751, 10.5513)
  line L673 (37.4751, 10.5513) -> (38.6464, 12.5801)
  line L674 (24.4741, -18.8337) -> (25.6454, -16.8049)
  line L675 (25.6454, -16.8049) -> (27.9882, -16.8049)
  line L676 (27.9882, -16.8049) -> (29.1594, -18.8337)
  line L677 (38.8144, -2.0645) -> (37.6431, -0.0357)
  line L678 (37.6431, -0.0357) -> (38.8144, 1.9931)
  line L679 (38.7554, 3.1855) -> (37.5841, 5.2143)
  line L680 (37.5841, 5.2143) -> (38.7554, 7.2431)
  line L681 (38.9794, -7.3885) -> (37.8081, -5.3597)
  line L682 (37.8081, -5.3597) -> (38.9794, -3.3309)
  line L683 (39.0884, -12.7245) -> (37.9171, -10.6957)
  line L684 (37.9171, -10.6957) -> (39.0884, -8.6669)
  line L685 (39.1484, -17.9755) -> (37.9771, -15.9467)
  line L686 (37.9771, -15.9467) -> (39.1484, -13.9179)
  line L687 (33.4991, -18.8087) -> (34.6704, -16.7799)
  line L688 (34.6704, -16.7799) -> (37.0132, -16.7799)
  line L689 (37.0132, -16.7799) -> (38.1844, -18.8087)
  line L690 (-22.0409, 15.6543) -> (-23.2121, 13.6255)
  line L691 (-23.2121, 13.6255) -> (-25.5549, 13.6255)
  line L692 (-25.5549, 13.6255) -> (-26.7262, 15.6543)
  line L693 (-32.0764, 6.9181) -> (-30.9052, 4.8893)
  line L694 (-30.9052, 4.8893) -> (-32.0764, 2.8605)
  line L695 (-32.1858, 12.2551) -> (-31.0146, 10.2263)
  line L696 (-31.0146, 10.2263) -> (-32.1858, 8.1975)
  line L697 (2.7374, -19.4429) -> (5.0802, -19.4429)
  line L698 (12.0554, -19.3999) -> (14.3982, -19.3999)
  line L699 (21.1504, -19.3709) -> (23.4932, -19.3709)
  line L700 (-35.2208, -8.3987) -> (-36.392, -10.4275)
  line L701 (-36.1617, -17.1049) -> (-34.9905, -19.1337)
  line L702 (-9.2774, 10.8355) -> (-11.6202, 10.8355)
  line L703 (-8.1062, 12.8643) -> (-9.2774, 10.8355)
  line L704 (-9.2774, 14.8931) -> (-8.1062, 12.8643)
  line L705 (-11.6202, 10.8355) -> (-12.7915, 12.8643)
  line L706 (-12.7915, 12.8643) -> (-11.6202, 14.8931)
  line L707 (-11.6202, 14.8931) -> (-9.2774, 14.8931)
  line L708 (13.4852, 24.4265) -> (11.1424, 24.4265)
  line L709 (27.2882, 16.5815) -> (24.9454, 16.5815)
  line L710 (36.3132, 16.6065) -> (33.9704, 16.6065)
  line L711 (38.5254, 13.9215) -> (37.3541, 15.9503)
  line L712 (30.1744, -19.3459) -> (32.5172, -19.3459)
  line L713 (4.1672, 24.3835) -> (1.8244, 24.3835)
  line L714 (-4.9278, 24.3545) -> (-7.2706, 24.3545)
  line L715 (-18.4488, 16.3535) -> (-20.7916, 16.3535)
  line L716 (-27.7672, 16.3105) -> (-30.11, 16.3105)
  line L717 (-31.1355, 15.6253) -> (-32.3067, 13.5965)
  line L718 (38.8144, -18.445) -> (-31.7211, -18.445)
  line L719 (-31.7211, -18.445) -> (-31.7211, 14.6109)
  line L720 (-12.475, 22.6532) -> (20.0445, 22.6532)
  line L721 (38.8144, 14.4269) -> (38.8144, -18.445)
  line L722 (18.6466, 14.4269) -> (36.1466, 14.4269)
  line L723 (20.0445, 22.6532) -> (19.4229, 22.6532)
  line L724 (19.4229, 22.6532) -> (19.4229, 14.4269)
  line L725 (19.4229, 14.4269) -> (38.8144, 14.4269)
  line L726 (-28.8534, 14.4269) -> (-11.3534, 14.4269)
  line L727 (-12.475, 22.6532) -> (-11.8894, 22.6532)
  line L728 (-11.8894, 22.6532) -> (-11.8894, 14.4269)
  line L729 (-11.8894, 14.4269) -> (-31.7211, 14.4269)
  line L730 (-31.7211, 14.4269) -> (-31.7211, 14.6109)
  line L731 (-11.8894, 22.6532) -> (19.4229, 22.6532)
  line L732 (19.4229, 22.6532) -> (19.4229, -18.445)
  line L733 (19.4229, -18.445) -> (-11.8894, -18.445)
  line L734 (-11.8894, -18.445) -> (-11.8894, 22.6532)
  line L735 (3.7668, 22.6532) -> (3.7668, -26.366)
  point P0 (0, 0)
  dimension "d58" = 30
  constraints: 1468 end point, 14 point on line, 5 midpoint, 2 parallel, 1 centre point, 1 horizontal, 1 perpendicular, 1 vertical
  measures "d58" diameter of A0
extrude "Wyciągnięcie proste10" cut sketch "Szkic15" against normal blind 3 contours L75 L76 L77 L78 L79 L80 | L146 L145 L144 L143 L142 L141 | L147 L148 L149 L150 L151 L152 | L158 L157 L156 L155 L154 L153 | L219 L220 L221 L222 L223 L224 | L230 L229 L228 L227 L226 L225 | L236 L235 L234 L233 L232 L231 | L249 L250 L251 L252 L253 L254 | L260 L259 L258 L257 L256 L255 | L266 L265 L264 L263 L262 L261 | L272 L271 L270 L269 L268 L267 | L273 L274 L275 L276 L277 L278 | L284 L283 L282 L281 L280 L279 | L285 L286 L287 L288 L289 L290 | L291 L292 L293 L294 L295 L296 | L297 L298 L299 L300 L301 L302 | L308 L307 L306 L305 L304 L303 | L314 L313 L312 L311 L310 L309 | L352 L353 L354 L355 L356 L357 | L375 L374 L373 L372 L371 L370 | L423 L422 L421 L420 L419 L418 | L441 L440 L439 L438 L437 L436 | L454 L455 L456 L457 L458 L459 | L465 L464 L463 L462 L461 L460 | L471 L470 L469 L468 L467 L466 | L472 L473 L474 L475 L476 L477 | L478 L479 L480 L481 L482 L483 | L490 L491 L492 L493 L494 L495 | L501 L500 L499 L498 L497 L496 | L502 L503 L504 L505 L506 L507 | L508 L509 L510 L511 L512 L513 | L519 L518 L517 L516 L515 L514 | L520 L521 L522 L523 L524 L525 | L597 L596 L595 L594 L593 L592 | L603 L602 L601 L600 L599 L598 | L609 L608 L607 L606 L605 L604 | L615 L614 L613 L612 L611 L610 | L621 L620 L619 L618 L617 L616
sketch "Szkic16" plane through (-32.7454, 17.1956, -2) normal (0, 0, -1) x (-1, 0, 0)
  arc A0 (0, 0) -> (0, -1.8) centre (0, -0.9) ccw projected
  line L0 (0, -0.9) -> (4.5, -0.9) construction
  line L1 (4.5, -1.8) -> (0, -1.8) projected
  line L2 (0, -1.5) -> (4.5, -1.5)
  line L3 (4.5, -0.3) -> (0, -0.3)
  arc A1 (0, -0.3) -> (0, -1.5) centre (0, -0.9) ccw
  arc A2 (4.5, -1.5) -> (4.5, -0.3) centre (4.5, -0.9) ccw
  line L4 (0, -0.9) -> (4.5, -0.9) construction
  line L5 (0, -1.8) -> (4.5, -1.8)
  line L6 (4.5, 0) -> (0, 0)
  arc A3 (0, 0) -> (0, -1.8) centre (0, -0.9) ccw
  arc A4 (4.5, -1.8) -> (4.5, 0) centre (4.5, -0.9) ccw
  arc A5 (9.4, -4.9) -> (7.6, -4.9) centre (8.5, -4.9) ccw projected
  arc A6 (7.6, -9.4) -> (9.4, -9.4) centre (8.5, -9.4) ccw projected
  line L7 (8.5, -4.9) -> (8.5, -9.4) construction
  line L8 (7.9, -4.9) -> (7.9, -9.4)
  line L9 (9.1, -9.4) -> (9.1, -4.9)
  arc A7 (9.1, -4.9) -> (7.9, -4.9) centre (8.5, -4.9) ccw
  arc A8 (7.9, -9.4) -> (9.1, -9.4) centre (8.5, -9.4) ccw
  line L10 (8.5, -9.4) -> (8.5, -4.9) construction
  line L11 (9.4, -9.4) -> (9.4, -4.9)
  line L12 (7.6, -4.9) -> (7.6, -9.4)
  arc A9 (7.6, -9.4) -> (9.4, -9.4) centre (8.5, -9.4) ccw
  arc A10 (9.4, -4.9) -> (7.6, -4.9) centre (8.5, -4.9) ccw
  line L13 (-33.69, 6.85) -> (-24.31, 6.85) projected
  line L14 (-29, 6.85) -> (-29, 3.0576)
  line L15 (8.5, -12.4) -> (8.5, -24.4) projected
  line L16 (8.5, -18.4) -> (5.4, -18.4)
  arc A11 (0, -35) -> (0, -36.8) centre (0, -35.9) ccw
  line L17 (0, -35.9) -> (4.5, -35.9) construction
  line L18 (4.5, -35) -> (0, -35)
  line L19 (0, -35.3) -> (4.5, -35.3)
  line L20 (4.5, -36.5) -> (0, -36.5)
  arc A12 (0, -35.3) -> (0, -36.5) centre (0, -35.9) ccw
  arc A13 (4.5, -36.5) -> (4.5, -35.3) centre (4.5, -35.9) ccw
  line L21 (0, -35.9) -> (4.5, -35.9) construction
  line L22 (0, -35) -> (4.5, -35)
  line L23 (4.5, -36.8) -> (0, -36.8)
  arc A14 (0, -35) -> (0, -36.8) centre (0, -35.9) ccw
  arc A15 (4.5, -36.8) -> (4.5, -35) centre (4.5, -35.9) ccw
  arc A16 (7.6, -31.9) -> (9.4, -31.9) centre (8.5, -31.9) ccw
  arc A17 (9.4, -27.4) -> (7.6, -27.4) centre (8.5, -27.4) ccw
  line L24 (8.5, -31.9) -> (8.5, -27.4) construction
  line L25 (7.9, -31.9) -> (7.9, -27.4)
  line L26 (9.1, -27.4) -> (9.1, -31.9)
  arc A18 (7.9, -31.9) -> (9.1, -31.9) centre (8.5, -31.9) ccw
  arc A19 (9.1, -27.4) -> (7.9, -27.4) centre (8.5, -27.4) ccw
  line L27 (8.5, -27.4) -> (8.5, -31.9) construction
  line L28 (9.4, -27.4) -> (9.4, -31.9)
  line L29 (7.6, -31.9) -> (7.6, -27.4)
  arc A20 (9.4, -27.4) -> (7.6, -27.4) centre (8.5, -27.4) ccw
  arc A21 (7.6, -31.9) -> (9.4, -31.9) centre (8.5, -31.9) ccw
  arc A22 (-58, -1.8) -> (-58, 0) centre (-58, -0.9) ccw
  line L30 (-58, -0.9) -> (-62.5, -0.9) construction
  line L31 (-62.5, -1.8) -> (-58, -1.8)
  line L32 (-58, -1.5) -> (-62.5, -1.5)
  line L33 (-62.5, -0.3) -> (-58, -0.3)
  arc A23 (-58, -1.5) -> (-58, -0.3) centre (-58, -0.9) ccw
  arc A24 (-62.5, -0.3) -> (-62.5, -1.5) centre (-62.5, -0.9) ccw
  line L34 (-58, -0.9) -> (-62.5, -0.9) construction
  line L35 (-58, -1.8) -> (-62.5, -1.8)
  line L36 (-62.5, 0) -> (-58, 0)
  arc A25 (-58, -1.8) -> (-58, 0) centre (-58, -0.9) ccw
  arc A26 (-62.5, 0) -> (-62.5, -1.8) centre (-62.5, -0.9) ccw
  arc A27 (-65.6, -4.9) -> (-67.4, -4.9) centre (-66.5, -4.9) ccw
  arc A28 (-67.4, -9.4) -> (-65.6, -9.4) centre (-66.5, -9.4) ccw
  line L37 (-66.5, -4.9) -> (-66.5, -9.4) construction
  line L38 (-65.9, -4.9) -> (-65.9, -9.4)
  line L39 (-67.1, -9.4) -> (-67.1, -4.9)
  arc A29 (-65.9, -4.9) -> (-67.1, -4.9) centre (-66.5, -4.9) ccw
  arc A30 (-67.1, -9.4) -> (-65.9, -9.4) centre (-66.5, -9.4) ccw
  line L40 (-66.5, -9.4) -> (-66.5, -4.9) construction
  line L41 (-67.4, -9.4) -> (-67.4, -4.9)
  line L42 (-65.6, -4.9) -> (-65.6, -9.4)
  arc A31 (-67.4, -9.4) -> (-65.6, -9.4) centre (-66.5, -9.4) ccw
  arc A32 (-65.6, -4.9) -> (-67.4, -4.9) centre (-66.5, -4.9) ccw
  arc A33 (-58, -36.8) -> (-58, -35) centre (-58, -35.9) ccw
  line L43 (-58, -35.9) -> (-62.5, -35.9) construction
  line L44 (-62.5, -35) -> (-58, -35)
  line L45 (-58, -35.3) -> (-62.5, -35.3)
  line L46 (-62.5, -36.5) -> (-58, -36.5)
  arc A34 (-58, -36.5) -> (-58, -35.3) centre (-58, -35.9) ccw
  arc A35 (-62.5, -35.3) -> (-62.5, -36.5) centre (-62.5, -35.9) ccw
  arc A36 (-62.5, -35) -> (-62.5, -36.8) centre (-62.5, -35.9) ccw
  line L47 (-58, -35) -> (-62.5, -35)
  line L48 (-58, -35.9) -> (-62.5, -35.9) construction
  line L49 (-62.5, -36.8) -> (-58, -36.8)
  arc A37 (-58, -36.8) -> (-58, -35) centre (-58, -35.9) ccw
  arc A38 (-67.1, -31.9) -> (-65.9, -31.9) centre (-66.5, -31.9) ccw
  arc A39 (-67.4, -31.9) -> (-65.6, -31.9) centre (-66.5, -31.9) ccw
  arc A40 (-67.4, -31.9) -> (-65.6, -31.9) centre (-66.5, -31.9) ccw
  line L50 (-65.6, -31.9) -> (-65.6, -27.4)
  line L51 (-65.9, -31.9) -> (-65.9, -27.4)
  line L52 (-66.5, -31.9) -> (-66.5, -27.4) construction
  line L53 (-66.5, -27.4) -> (-66.5, -31.9) construction
  line L54 (-67.1, -27.4) -> (-67.1, -31.9)
  line L55 (-67.4, -27.4) -> (-67.4, -31.9)
  arc A41 (-65.9, -27.4) -> (-67.1, -27.4) centre (-66.5, -27.4) ccw
  arc A42 (-65.6, -27.4) -> (-67.4, -27.4) centre (-66.5, -27.4) ccw
  arc A43 (-65.6, -27.4) -> (-67.4, -27.4) centre (-66.5, -27.4) ccw
  point P0 (-32.7454, -17.1956)
  point P1 (2.25, -0.9)
  point P2 (2.25, -0.9)
  point P3 (8.5, -7.15)
  point P4 (8.5, -7.15)
  point P5 (2.25, -35.9)
  point P6 (2.25, -35.9)
  point P7 (8.5, -29.65)
  point P8 (8.5, -29.65)
  point P9 (-60.25, -0.9)
  point P10 (-60.25, -0.9)
  point P11 (-66.5, -7.15)
  point P12 (-66.5, -7.15)
  point P13 (-60.25, -35.9)
  point P14 (-60.25, -35.9)
  point P15 (-66.5, -29.65)
  point P16 (-66.5, -29.65)
  point P17 (-58, 0)
  point P18 (-62.5, -1.8)
  point P19 (-65.6, -31.9)
  point P20 (-67.4, -31.9)
  point P21 (-58, -36.8)
  point P22 (0, -36.8)
  point P23 (4.5, -35)
  point P24 (9.4, -31.9)
  point P25 (7.6, -4.9)
  point P26 (7.6, -9.4)
  dimension "d61" = 1.2
  dimension "d62" = 1.2
  constraints: 138 end point, 93 symmetric about line, 82 point on circle, 41 centre point, 16 tangent, 7 equal length, 6 midpoint, 2 vertical, 1 horizontal, 33 other
  measures "d61" diameter of A2
  measures "d62" diameter of A8
extrude "Wyciągnięcie proste11" cut sketch "Szkic16" against normal blind 2
fillet "Zaokrąglenie1" radius 0.6 32 edges at (24.6546, 16.2956, -2) (27.5046, 16.8956, -2) (30.3546, 16.2956, -2) (27.5046, 15.6956, -2) (33.7546, 12.8956, -2) (34.3546, 10.0456, -2) (33.7546, 7.1956, -2) (33.1546, 10.0456, -2) (33.7546, -9.6044, -2) (34.3546, -12.4544, -2) (33.7546, -15.3044, -2) (33.1546, -12.4544, -2) (24.6546, -18.7044, -2) (27.5046, -18.1044, -2) (30.3546, -18.7044, -2) (27.5046, -19.3044, -2) (-37.8454, -18.7044, -2) (-34.9954, -18.1044, -2) (-32.1454, -18.7044, -2) (-34.9954, -19.3044, -2) (-41.2454, -9.6044, -2) (-40.6454, -12.4544, -2) (-41.2454, -15.3044, -2) (-41.8454, -12.4544, -2) (-41.2454, 12.8956, -2) (-40.6454, 10.0456, -2) (-41.2454, 7.1956, -2) (-41.8454, 10.0456, -2) (-37.8454, 16.2956, -2) (-34.9954, 16.8956, -2) (-32.1454, 16.2956, -2) (-34.9954, 15.6956, -2)
sketch "Szkic17" plane through (0, 0, 0) normal (0, 0, -1) x (-1, 0, 0)
  arc A0 (-31.7546, 18.2956) -> (-35.7546, 14.2956) centre (-31.7546, 14.2956) ccw projected
  line L0 (39.2454, 11.2956) -> (39.2454, -13.7044)
  line L1 (36.2454, -16.7044) -> (-28.7546, -16.7044)
  line L2 (-31.7546, -13.7044) -> (-31.7546, 11.2956)
  line L3 (-13.2546, 18.2956) -> (-13.2546, 21.2956) projected
  line L4 (-13.2546, 18.2956) -> (-9.2546, 18.2956) construction
  line L5 (16.7454, 16.2956) -> (16.7454, 21.2956)
  line L6 (13.7454, 24.2956) -> (-6.2546, 24.2956)
  line L7 (-9.2546, 21.2956) -> (-9.2546, 16.2956)
  line L8 (-28.7546, 14.2956) -> (-11.2546, 14.2956)
  line L9 (18.7454, 14.2956) -> (36.2454, 14.2956)
  arc A1 (-28.7546, 14.2956) -> (-31.7546, 11.2956) centre (-28.7546, 11.2956) ccw
  arc A2 (-6.2546, 24.2956) -> (-9.2546, 21.2956) centre (-6.2546, 21.2956) ccw
  arc A3 (16.7454, 21.2956) -> (13.7454, 24.2956) centre (13.7454, 21.2956) ccw
  arc A4 (39.2454, 11.2956) -> (36.2454, 14.2956) centre (36.2454, 11.2956) ccw
  arc A5 (36.2454, -16.7044) -> (39.2454, -13.7044) centre (36.2454, -13.7044) ccw
  arc A6 (-31.7546, -13.7044) -> (-28.7546, -16.7044) centre (-28.7546, -13.7044) ccw
  arc A7 (-11.2546, 14.2956) -> (-9.2546, 16.2956) centre (-11.2546, 16.2956) ccw
  arc A8 (16.7454, 16.2956) -> (18.7454, 14.2956) centre (18.7454, 16.2956) ccw
  point P0 (0, 0)
  point P1 (39.2454, -16.7044)
  point P2 (39.2454, 14.2956)
  point P3 (-31.7546, -16.7044)
  dimension "d68" = 71
  dimension "d69" = 31
  dimension "d74" = 3
  dimension "d75" = 2
  constraints: 18 end point, 16 point on circle, 16 tangent, 8 centre point, 8 point on line, 6 equal radius, 4 parallel, 3 horizontal, 2 perpendicular
  measures "d68" distance of point (39.245, -16.704) point (-31.755, -16.704)
  measures "d69" distance of point (39.245, 14.296) point (39.245, -16.704)
  measures "d74" radius of A1
  measures "d75" radius of A7
extrude "Wyciągnięcie proste12" cut sketch "Szkic17" against normal blind 0.5
chamfer "Faza4" distance 0.25 angle 45 4 edges at (-3.7525, -16.7044, -4) (-3.7525, -18.7044, -4) (-3.7454, 25.2956, -3.5) (-3.7454, 24.2956, -3.5)
